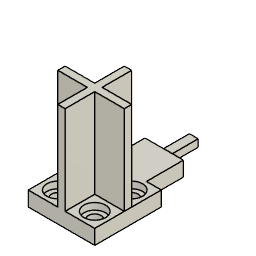
LDR Platform (Autodesk Fusion 360 design; units mm, degrees)
Autodesk Fusion 360 part; units mm, degrees
sketch "Sketch1" plane through (0, 0, 0) normal (0, 0, 1) x (1, 0, 0)
  line L0 (-1, 10) -> (5, 10)
  line L1 (5, 10) -> (5, -10)
  line L2 (5, -10) -> (-1, -10)
  line L3 (-1, -10) -> (-1, 10)
  line L4 (-1, -10) -> (-11, -10)
  line L5 (5, -10) -> (15, -10)
  line L6 (-11, -10) -> (-11, -35)
  line L7 (15, -10) -> (15, -35)
  line L8 (-11, -35) -> (-20, -35)
  line L9 (-20, -35) -> (-20, -80)
  line L10 (15, -35) -> (25, -35)
  line L11 (-20, -80) -> (25, -80)
  line L12 (25, -80) -> (25, -35)
  dimension "d1" = 20
  dimension "d2" = 10
  dimension "d3" = 6
  dimension "d4" = 10
  dimension "d5" = 45
  constraint horizontal L0
  constraint vertical L1
  constraint horizontal L2
  constraint vertical L3
  constraint perpendicular L3 L4
  constraint perpendicular L1 L5
  constraint perpendicular L4 L6
  constraint perpendicular L5 L7
  constraint perpendicular L6 L8
  constraint perpendicular L5 L9
  constraint perpendicular L7 L10
  constraint perpendicular L9 L11
  measures "d1" distance of L0.end L1.end
  measures "d2" distance of L2.end L4.end
  measures "d3" distance of L1.end L2.end
  measures "d4" distance of L1.end L5.end
  measures "d5" distance of L8.end L9.end
extrude "Extrude1" add sketch "Sketch1" along normal blind 5 contours L0 L1 L2 L3
sketch "Sketch2" plane through (0, 0, 5) normal (0, 0, 1) x (-1, 0, 0)
  line L0 (-5, 10) -> (-5, -10)
  line L1 (-5, -10) -> (1, -10)
  line L2 (1, -10) -> (1, 10)
  line L3 (-25, 55) -> (-25, 60)
  line L4 (-25, 60) -> (20, 60)
  line L5 (20, 55) -> (-25, 55)
  line L6 (-2.5, 35) -> (-5, 35)
  line L7 (-5, 35) -> (-5, 80)
  line L8 (-2.5, 35) -> (0, 35)
  line L9 (0, 35) -> (0, 80)
  line L10 (1, 10) -> (-5, 10)
  line L11 (-5, 80) -> (-2.5, 80)
  line L12 (0, 80) -> (-2.5, 80)
  line L13 (20, 60) -> (19.7373, 60)
  line L14 (20, 55) -> (20, 57.5)
  line L15 (20, 60) -> (20, 57.5)
  constraint perpendicular L3 L5
  constraint coincident L4 L13.end
extrude "Extrude2" add sketch "Sketch1" along normal blind 7.5 contours L2 L4 L5 L6 L7 L8 L9 L10 L11 L12
extrude "Extrude3" add sketch "Sketch1" against normal blind 2.5 contours L2 L4 L5 L6 L7 L8 L9 L10 L11 L12
extrude "Extrude4" add sketch "Sketch2" along normal blind 62.6 contours L3 L4 L5 L7 | L4 L5 L7 L9 | L5 L6 L7 L8 L9 | L4 L7 L9 L11 L12 | L4 L5 L9 L13 L14 L15
sketch "Sketch3" plane through (0, 0, 7.5) normal (0, 0, 1) x (-1, 0, 0)
  line L0 (20, 55) -> (0, 55)
  line L1 (0, 55) -> (0, 35)
  line L2 (0, 35) -> (-5, 35)
  line L3 (-5, 35) -> (-5, 55)
  line L4 (-5, 55) -> (-25, 55)
  line L5 (-25, 55) -> (-25, 35)
  line L6 (-25, 35) -> (-15, 35)
  line L7 (-15, 35) -> (-15, 10)
  line L8 (-15, 10) -> (11, 10)
  line L9 (11, 10) -> (11, 35)
  line L10 (11, 35) -> (20, 35)
  line L11 (20, 35) -> (20, 55)
  circle A0 centre (-15, 45) radius 7.35
  circle A1 centre (-15, 70) radius 7.35
  circle A2 centre (10, 70) radius 7.35
  circle A3 centre (10, 45) radius 7.35
  line L12 (0, 80) -> (0, 60)
  line L13 (0, 60) -> (20, 60)
  line L14 (-5, 60) -> (-5, 80)
  line L15 (-25, 60) -> (-5, 60)
  dimension "d15" = 10
  dimension "d16" = 10
  dimension "d17" = 10
  dimension "d18" = 10
  dimension "d19" = 10
  dimension "d20" = 10
  dimension "d21" = 10
  dimension "d22" = 10
  dimension "d23" = 14.7
  dimension "d24" = 14.7
  dimension "d25" = 14.7
  dimension "d26" = 14.7
  measures "d15" distance of L4 A0.centre
  measures "d16" distance of L3 A0.centre
  measures "d17" distance of L0 A3.centre
  measures "d18" distance of L1 A3.centre
  measures "d19" distance of A2.centre L12
  measures "d20" distance of A2.centre L13
  measures "d21" distance of A1.centre L14
  measures "d22" distance of A1.centre L15
  measures "d23" diameter of A1
  measures "d24" diameter of A2
  measures "d25" diameter of A3
  measures "d26" diameter of A0
extrude "Extrude5" cut sketch "Sketch3" against normal blind 4.5 contours A0 | A1 | A2 | A3
sketch "Sketch4" plane through (0, 0, 3) normal (0, 0, 1) x (-1, 0, 0)
  circle A0 centre (-15, 45) radius 7.35
  circle A1 centre (-15, 70) radius 4.25
  circle A2 centre (10, 70) radius 4.25
  circle A3 centre (10, 45) radius 4.25
  circle A4 centre (-15, 45) radius 4.25
  line L0 (0, 60) -> (20, 60)
  dimension "d29" = 10
  dimension "d30" = 8.5
  dimension "d31" = 8.5
  dimension "d32" = 8.5
  dimension "d33" = 8.5
  constraint concentric A0 A4
  measures "d29" distance of A2.centre L0
  measures "d30" diameter of A4
  measures "d31" diameter of A3
  measures "d32" diameter of A2
  measures "d33" diameter of A1
extrude "Extrude6" cut sketch "Sketch4" against normal blind 6 contours A1 | A2 | A3 | A4
